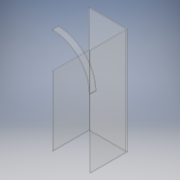
# Autodesk Inventor part: Sorter
Saved by Autodesk Inventor 2019 (Build 230136000, 136)
## iProperties
Created: 2018-11-20
Part Number: Sorter
Material: Polycarbonate, Clear
Document SubType Name: Modeling
Designer: User
Density: 1.2 g/cm^3
Appearance: Polycarbonate - Clear
Author: User
Autodesk Inventor part; units mm, degrees
ref_plane "YZ Plane" through (0, 0, 0) normal (1, 0, 0) x (0, 1, 0)
ref_plane "XZ Plane" through (0, 0, 0) normal (0, 1, 0) x (-1, 0, 0)
ref_plane "XY Plane" through (0, 0, 0) normal (0, 0, 1) x (1, 0, 0)
sketch "Sketch1" plane through (0, 0, 0) normal (0, 0, 1) x (1, 0, 0)
  line L0 (0, 0) -> (79.9084, 0)
  line L1 (79.9084, 0) -> (79.9084, 219.6084)
  line L2 (79.9084, 219.6084) -> (0, 219.6084)
  line L3 (0, 219.6084) -> (0, 0)
  dimension "d0" = 79.9084
  dimension "d1" = 219.6084
  constraints: 8 end point, 2 parallel, 1 horizontal, 1 perpendicular
  measures "d0" distance of L2.end L1.end
  measures "d1" distance between parallel lines of L2 L0
extrude "Extrusion1" add sketch "Sketch1" along normal blind 76.2
sketch "Sketch2" plane through (0, 0, 0) normal (0, -1, 0) x (1, 0, 0)
  line L0 (79.9084, 0) -> (79.9084, 76.2) projected
  line L1 (0, 0) -> (79.9084, 0) projected
  line L2 (0, 76.2) -> (79.9084, 76.2) projected
  line L3 (78.0542, 1.8542) -> (1.8542, 1.8542)
  line L4 (1.8542, 1.8542) -> (1.8542, 76.2)
  line L5 (1.8542, 76.2) -> (78.0542, 76.2)
  line L6 (78.0542, 76.2) -> (78.0542, 1.8542)
  dimension "d4" = 1.8542
  dimension "d5" = 1.8542
  dimension "d6" = 76.2
  constraints: 8 end point, 2 parallel, 1 horizontal, 1 perpendicular, 1 point on line
  measures "d4" distance from line of L0 L3.start
  measures "d5" distance from line of L1 L3.start
  measures "d6" distance of L4.end L5.end
extrude "Extrusion2" cut sketch "Sketch2" against normal blind 228.6
sketch "Sketch3" plane through (0, 0, 76.2) normal (0, 0, 1) x (1, 0, 0)
  line L0 (1.8542, 0) -> (1.8542, 219.6084) projected
  line L1 (0, 219.6084) -> (1.8542, 219.6084)
  line L2 (1.8542, 219.6084) -> (1.8542, 143.4084)
  line L3 (1.8542, 143.4084) -> (0, 143.4084)
  line L4 (0, 143.4084) -> (0, 219.6084)
  point P0 (0, 0)
  dimension "d9" = 76.2
  constraints: 8 end point, 2 parallel, 1 horizontal, 1 perpendicular, 1 point on line
  measures "d9" distance of L1.end L2.end
extrude "Extrusion3" cut sketch "Sketch3" against normal blind 74.3458
sketch "Sketch9" plane through (0, 0, 76.2) normal (0, 0, 1) x (1, 0, 0)
  line L0 (78.0542, 219.6084) -> (78.0542, 0) projected
  line L1 (0, 143.4084) -> (0, 219.6084) projected
  arc A0 (78.0542, 139.6114) -> (0, 217.6656) centre (0.5141, 140.1255) ccw
  line L2 (0, 217.6656) -> (78.0542, 139.6114) construction
  line L3 (0, 217.6656) -> (110.3853, 217.6656) construction
  line L4 (78.0542, 139.6114) -> (76.2, 139.6114)
  line L5 (0, 217.6656) -> (0, 215.8114)
  arc A1 (76.2, 139.6114) -> (0, 215.8114) centre (0.257, 139.8685) ccw
  point P0 (0, 0)
  dimension "d22" = 45
  dimension "d23" = 1.8542
  dimension "d24" = 1.8542
  constraints: 8 end point, 4 point on circle, 2 centre point, 2 horizontal, 2 point on line, 1 equal length
  measures "d22" angle of L2 L3
  measures "d23" distance of L2.end L4.end
  measures "d24" distance of L2.start L5.end
extrude "Extrusion7" add sketch "Sketch9" against normal blind 12.7
body "Solid1"
